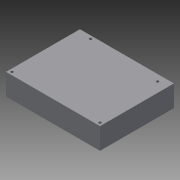
# Autodesk Inventor part: udoomountingholes
Saved by Autodesk Inventor 2015 (Build 190159000, 159)
## iProperties
Created: 2014-11-13
Part Number: udoomountingholes
Material: Generic
Document SubType Name: Modeling
Designer: ericd_000
Density: 1 g/cm^3
Appearance: Default
Author: ericd_000
Autodesk Inventor part; units mm, degrees
ref_plane "YZ Plane" through (0, 0, 0) normal (1, 0, 0) x (0, 1, 0)
ref_plane "XZ Plane" through (0, 0, 0) normal (0, 1, 0) x (-1, 0, 0)
ref_plane "XY Plane" through (0, 0, 0) normal (0, 0, 1) x (1, 0, 0)
sketch "Sketch1" plane through (0, 0, 0) normal (0, 0, 1) x (1, 0, 0)
  line L0 (-55, 43.25) -> (55, 43.25)
  line L1 (55, 43.25) -> (55, -43.25)
  line L2 (55, -43.25) -> (-55, -43.25)
  line L3 (-55, -43.25) -> (-55, 43.25)
  circle A0 centre (-39, 39.75) radius 1.55
  circle A1 centre (-51.5, -39.75) radius 1.55
  circle A2 centre (43.5, 35.75) radius 1.55
  circle A3 centre (51.5, -39.75) radius 1.55
  point P0 (0, 0)
  point P1 (-55, 0)
  point P2 (0, 43.25)
  dimension "d0" = 110
  dimension "d1" = 86.5
  dimension "d2" = 16
  dimension "d3" = 83
  dimension "d4" = 3.5
  dimension "d5" = 3.5
  dimension "d6" = 98.5
  dimension "d7" = 79
  dimension "d8" = 106.5
  dimension "d9" = 3.5
  dimension "d10" = 3.1
  dimension "d11" = 3.1
  dimension "d12" = 3.1
  dimension "d13" = 3.1
  constraints: 8 end point, 4 centre point, 2 midpoint, 2 parallel, 1 horizontal, 1 horizontal alignment, 1 perpendicular, 1 vertical alignment
  measures "d0" distance of L0.start L0.end
  measures "d1" distance of L2.end L0.start
  measures "d2" distance from line of L3 A0.centre
  measures "d3" distance from line of L2 A0.centre
  measures "d4" distance from line of L3 A1.centre
  measures "d5" distance from line of A1.centre L2
  measures "d6" distance from line of L3 A2.centre
  measures "d7" distance from line of L2 A2.centre
  measures "d8" distance from line of L3 A3.centre
  measures "d9" distance from line of L2 A3.centre
  measures "d10" diameter of A3
  measures "d11" diameter of A1
  measures "d12" diameter of A0
  measures "d13" diameter of A2
extrude "Extrusion1" add sketch "Sketch1" along normal blind 25
body "Solid1"
